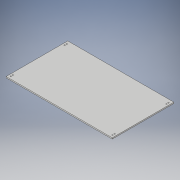
# Autodesk Inventor part: Plexiglass base
Saved by Autodesk Inventor 2019 (Build 230136000, 136)
## iProperties
Created: 2019-02-04
Part Number: Plexiglass base
Material: Generic
Document SubType Name: Modeling
Designer: mrhftc
Density: 1 g/cm^3
Appearance: Default
Author: mrhftc
Autodesk Inventor part; units mm, degrees
ref_plane "YZ Plane" through (0, 0, 0) normal (1, 0, 0) x (0, 1, 0)
ref_plane "XZ Plane" through (0, 0, 0) normal (0, 1, 0) x (-1, 0, 0)
ref_plane "XY Plane" through (0, 0, 0) normal (0, 0, 1) x (1, 0, 0)
sketch "Sketch1" plane through (0, 0, 0) normal (0, 1, 0) x (-1, 0, 0)
  line L0 (108.5784, -54.8383) -> (-284.9486, -54.8383)
  line L1 (-284.9486, -54.8383) -> (-284.9486, -283.4383)
  line L2 (-284.9486, -283.4383) -> (108.5784, -283.4383)
  line L3 (108.5784, -283.4383) -> (108.5784, -54.8383)
  point P0 (0, 0)
  dimension "d0" = 393.527
  dimension "d1" = 228.6
  constraints: 8 end point, 2 parallel, 1 horizontal, 1 perpendicular
  measures "d0" distance between parallel lines of L1 L3
  measures "d1" distance between parallel lines of L0 L2
extrude "Extrusion1" add sketch "Sketch1" along normal blind 4.3688
sketch "Sketch2" plane through (0, 4.3688, 0) normal (0, 1, 0) x (1, 0, 0)
  line L0 (-108.5784, 54.8383) -> (284.9486, 54.8383) construction
  line L1 (284.9486, 54.8383) -> (284.9486, 283.4383) construction
  line L2 (284.9486, 283.4383) -> (-108.5784, 283.4383) construction
  line L3 (-108.5784, 283.4383) -> (-108.5784, 54.8383) construction
  line L4 (88.1851, 283.4383) -> (88.1851, 54.8383) construction
  line L5 (268.9486, 0) -> (284.9486, 0) construction
  line L6 (284.9486, 0) -> (284.9486, 336) construction
  line L7 (268.9486, 336) -> (284.9486, 336) construction
  line L8 (268.9486, 336) -> (268.9486, 0) construction
  circle A0 centre (276.9486, 64) radius 2
  circle A1 centre (276.9486, 72) radius 2
  circle A2 centre (276.9486, 264) radius 2
  circle A3 centre (276.9486, 272) radius 2
  circle A4 centre (-100.5784, 264) radius 2
  circle A5 centre (-100.5784, 72) radius 2
  circle A6 centre (-100.5784, 64) radius 2
  circle A7 centre (-100.5784, 272) radius 2
  dimension "d16" = 64
  dimension "d17" = 72
  dimension "d20" = 64
  dimension "d21" = 72
  dimension "d24" = 4
  dimension "d25" = 4
  dimension "d26" = 4
  dimension "d27" = 4
  dimension "d28" = 9.1617
  dimension "d29" = 17.1617
  dimension "d30" = 19.4383
  dimension "d31" = 11.4383
  dimension "d34" = 8
  dimension "d35" = 8
  dimension "d36" = 8
  dimension "d37" = 8
  dimension "d38" = 8
  constraints: 10 end point, 8 centre point, 4 symmetric about line, 2 parallel, 1 collinear, 1 midpoint, 4 other
  measures "d16" distance from line of L5 A0.centre
  measures "d17" distance from line of L5 A1.centre
  measures "d20" distance from line of L7 A3.centre
  measures "d21" distance from line of L7 A2.centre
  measures "d24" diameter of A2
  measures "d25" diameter of A3
  measures "d26" diameter of A0
  measures "d27" diameter of A1
  measures "d28" distance from line of L0 A0.centre
  measures "d29" distance from line of L0 A1.centre
  measures "d30" distance from line of L2 A2.centre
  measures "d31" distance from line of L2 A3.centre
  measures "d34" distance from line of L8 A1.centre
  measures "d35" distance from line of L1 A2.centre
  measures "d36" distance from line of L1 A3.centre
  measures "d37" distance from line of A1.centre L6
  measures "d38" distance from line of L6 A0.centre
extrude "Extrusion2" cut sketch "Sketch2" against normal up to next
body "Solid1"
